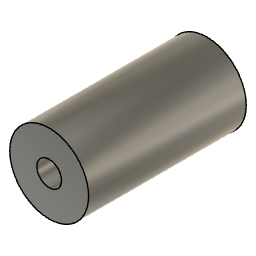
adaptador eje v1 (Autodesk Fusion 360 design; units mm, degrees)
Autodesk Fusion 360 part; units mm, degrees
sketch "Sketch1" plane through (0, 0, 0) normal (1, 0, 0) x (0, 1, 0)
  line L0 (0, 0) -> (30, 0)
  line L1 (30, 0) -> (30, 16.161)
  line L2 (30, 16.161) -> (0, 16.161)
  line L3 (0, 16.161) -> (0, 0)
  line L4 (15, 0) -> (15, 16.161)
  dimension "d1" = 30
  constraint horizontal L0
  constraint vertical L1
  constraint horizontal L2
  constraint vertical L3
  constraint coincident L0.start L3.end
  constraint midpoint L0 L4.start
  constraint midpoint L2 L4.end
  measures "d1" distance of L0.start L0.end
extrude "Extrude1" add sketch "Sketch1" along normal blind 25
sketch "Sketch2" plane through (0, 0, 0) normal (0, -1, 0) x (1, 0, 0)
  line L0 (0, 16.161) -> (0, 0)
  line L1 (0, 0) -> (25, 0)
  line L2 (25, 0) -> (25, 16.161)
  line L3 (25, 16.161) -> (0, 16.161)
  circle A0 centre (12.5, 8.0805) radius 2.35
  dimension "d4" = 4.7
  measures "d4" diameter of A0
sketch "Sketch3" plane through (0, 0, 0) normal (0, -1, 0) x (1, 0, 0)
sketch "Sketch4" plane through (0, 30, 0) normal (0, 1, 0) x (-1, 0, 0)
  line L0 (0, 0) -> (0, 16.161)
  line L1 (0, 16.161) -> (-25, 16.161)
  line L2 (-25, 16.161) -> (-25, 0)
  line L3 (-25, 0) -> (0, 0)
  circle A0 centre (-12.5, 8.0805) radius 2.4
  dimension "d5" = 4.8
  measures "d5" diameter of A0
extrude "Extrude2" cut sketch "Sketch4" against normal blind 10 contours A0
extrude "Extrude3" cut sketch "Sketch2" against normal blind 10 contours A0
sketch "Sketch5" plane through (0, 0, 0) normal (0, -1, 0) x (1, 0, 0)
  circle A0 centre (12.5, 8.0805) radius 2.35
  line L0 (0, 16.161) -> (0, 0)
  line L1 (0, 0) -> (25, 0)
  line L2 (25, 0) -> (25, 16.161)
  line L3 (25, 16.161) -> (0, 16.161)
  circle A1 centre (12.5, 8.0805) radius 7.5
  dimension "d10" = 15
  constraint concentric A0 A1
  measures "d10" diameter of A1
extrude "Extrude4" cut sketch "Sketch5" against normal blind 45 contours L0 L1 L2 L3
